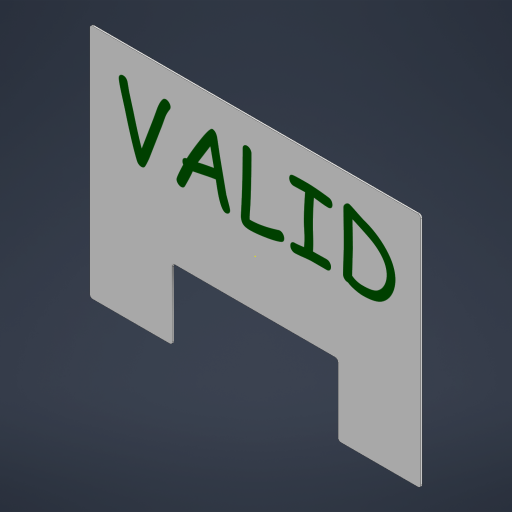
# Autodesk Inventor part: Blocker
Saved by Autodesk Inventor 2023 (Build 270158000, 158)
## iProperties
Created: 2023-10-24
Part Number: Blocker
Material: Generic
Document SubType Name: Modeling
Designer: diego
Density: 1 g/cm^3
Appearance: Default
Author: diego
Autodesk Inventor part; units mm, degrees
ref_plane "YZ Plane" through (0, 0, 0) normal (1, 0, 0) x (0, 1, 0)
ref_plane "XZ Plane" through (0, 0, 0) normal (0, 1, 0) x (-1, 0, 0)
ref_plane "XY Plane" through (0, 0, 0) normal (0, 0, 1) x (1, 0, 0)
sketch "Sketch2" plane through (0, 0, 0) normal (0, 0, 1) x (1, 0, 0)
  line L0 (-177.8, 127) -> (177.8, 127)
  line L1 (177.8, 127) -> (177.8, -127)
  line L2 (177.8, -127) -> (-177.8, -127)
  line L3 (-177.8, -127) -> (-177.8, 127)
  line L4 (-88.8917, -127) -> (-88.8917, 127)
  line L5 (88.9035, -127) -> (88.9035, 127)
  line L6 (-88.8917, -50.7948) -> (88.9035, -50.7948)
  point P0 (0, 0)
  dimension "d7" = 355.6
  dimension "d8" = 254
  dimension "d9" = 177.7952
  constraints: 14 end point, 6 point on line, 4 perpendicular, 2 parallel, 1 horizontal
  measures "d7" distance of L0.start L0.end
  measures "d8" distance of L2.end L0.start
  measures "d9" distance of L6.start L6.end
extrude "Extrusion1" add sketch "Sketch2" along normal blind 1.5875 contours L0 L4 L2 L3 | L0 L5 L6 L4 | L0 L1 L2 L5
fillet "Fillet1" radius 3.175 1 edges at (177.8, 127, 0.7937)
fillet "Fillet2" radius 3.175 1 edges at (177.8, -127, 0.7937)
fillet "Fillet3" radius 3.175 1 edges at (-177.8, 127, 0.7937)
fillet "Fillet4" radius 3.175 1 edges at (-177.8, -127, 0.7937)
fillet "Fillet5" radius 3.175 1 edges at (-88.8917, -127, 0.7937)
fillet "Fillet6" radius 3.175 1 edges at (-88.8917, -50.7948, 0.7937)
fillet "Fillet7" radius 3.175 1 edges at (88.9035, -50.7948, 0.7937)
fillet "Fillet8" radius 3.175 1 edges at (88.9035, -127, 0.7937)
sketch "Sketch4" plane through (0, 0, 1.5875) normal (0, 0, 1) x (1, 0, 0)
  line L0 (-166.9509, 119.7078) -> (168.8331, 119.7078) construction
  line L1 (168.8331, 119.7078) -> (168.8331, 0.7529) construction
  line L2 (168.8331, 0.7529) -> (-166.9509, 0.7529) construction
  line L3 (-166.9509, 0.7529) -> (-166.9509, 119.7078) construction
  point P0 (0, 0)
  constraints: 2 other
body "Solid1"
